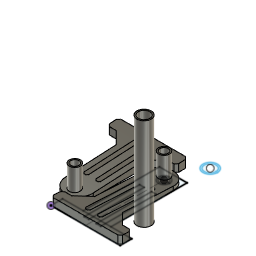
10lbs spool holder v3 (Autodesk Fusion 360 design; units mm, degrees)
Autodesk Fusion 360 part; units mm, degrees
sketch "Sketch1" plane through (0, 0, 0) normal (0, 0, 1) x (1, 0, 0) in component "Side"
  line L0 (0, 0) -> (150, 0)
  line L1 (75, 0) -> (75, 170) construction
  circle A0 centre (75, 170) radius 12
  circle A1 centre (75, 170) radius 9
  line L2 (150, 0) -> (150, 25)
  line L3 (0, 0) -> (0, 25)
  line L4 (0, 25) -> (150, 25)
  line L5 (45, 190) -> (105, 190)
  circle A2 centre (102.7681, 242.3233) radius 12.5
  circle A3 centre (102.7681, 242.3233) radius 15.5
  line L6 (45, 190) -> (45, 25)
  line L7 (105, 190) -> (105, 25)
  line L8 (57, 135) -> (67, 135)
  line L9 (67, 135) -> (67, 15)
  line L10 (67, 15) -> (57, 15)
  line L11 (57, 15) -> (57, 135)
  line L12 (93, 15) -> (93, 135)
  line L13 (93, 135) -> (83, 135)
  line L14 (83, 135) -> (83, 15)
  line L15 (83, 15) -> (93, 15)
  dimension "d1" = 150
  dimension "d2" = 170
  dimension "d3" = 24
  dimension "d4" = 18
  dimension "d5" = 25
  dimension "d6" = 25
  dimension "d9" = 60
  dimension "d10" = 190
  dimension "d11" = 25
  dimension "d16" = 25
  dimension "d17" = 31
  dimension "d20" = 45
  dimension "d28" = 10
  dimension "d29" = 120
  dimension "d30" = 15
  dimension "d31" = 8
  constraint coincident L0.start L3.start
  constraint horizontal L0
  constraint midpoint L0 L1.start
  constraint perpendicular L0 L1
  constraint coincident L1.end A0.centre
  constraint perpendicular L0 L2
  constraint perpendicular L0 L3
  constraint horizontal L4
  constraint perpendicular L1 L5
  constraint concentric A2 A3
  constraint coincident L4 L6.end
  constraint perpendicular L4 L6
  constraint coincident L4 L7.end
  constraint perpendicular L4 L7
  constraint horizontal L8
  constraint vertical L9
  constraint horizontal L10
  constraint vertical L11
  constraint symmetric L1 L8.start L12.end
  constraint symmetric L1 L8.end L13.end
  constraint symmetric L1 L9.end L14.end
  constraint symmetric L1 L10.end L12.start
  measures "d1" distance of L0.start L0.end
  measures "d2" distance of L1.start L1.end
  measures "d3" diameter of A0
  measures "d4" diameter of A1
  measures "d5" distance of L0.end L2.end
  measures "d6" distance of L0.start L3.end
  measures "d9" distance of L5.start L5.end
  measures "d10" distance of L0 L5
  measures "d11" distance of L0 L4
  measures "d16" diameter of A2
  measures "d17" diameter of A3
  measures "d20" distance of L3 L6
  measures "d28" distance of L8.start L8.end
  measures "d29" distance of L8.start L10.end
  measures "d30" distance of L0 L10
  measures "d31" distance of L1 L9
extrude "Extrude4" add sketch "Sketch1" along normal blind 10 contours L0 L2 L3 L4 L9 L10 L11 L12 L14 L15 | L4 L5 L6 L7 L8 L9 L11 L12 L13 L14 makes body 1 in component "Side"
draft "Draft1" angle -3 neutral plane through (93, 135, 0) pull (0, -1, 0) 1 faces at (15, 16.6667, 10) on bodies 1 in component "Side"
extrude "Extrude5" add sketch "Sketch1" along normal blind 55 contours A0 bodies 1 in component "Side"
chamfer "Chamfer1" distance 5 angle 45 4 edges at (0, 25, 7.8824) (0, 0, 8.5375) (150, 0, 8.5375) (150, 25, 7.8824) on bodies 1 in component "Side"
chamfer "Chamfer2" distance 25 angle 45 2 edges at (45, 25, 7.8824) (105, 25, 7.8824) on bodies 1 in component "Side"
fillet "Fillet1" radius 30 2 edges at (45, 190, 3.5588) (105, 190, 3.5588) on bodies 1 in component "Side"
chamfer "Chamfer3" distance 3 angle 45 8 edges at (93, 135, 5) (93, 15, 8.1445) (67, 15, 8.1445) (67, 135, 5) (83, 135, 5) (83, 15, 8.1445) (57, 15, 8.1445) (57, 135, 5) on bodies 1 in component "Side"
copy_body "CopyPasteBodies2" bodies 1 makes body 2 in component "Side"
move_body "Move2" bodies 2 to x (-1, 0, 0) y (0, -1, 0) z (0, 0, 1) at (76.008, 220.5643, 0) in component "Side"
extrude "Extrude6" add sketch "Sketch1" along normal blind 200 separate body contours A3 makes body 3 in component "Side"
move_body "Move3" bodies 3 to x (1, 0, 0) y (0, 1, 0) z (0, 0, 1) at (28.2686, -171.6106, 0) in component "Side"
extrude "Extrude1" [suppressed] in component "Side"
extrude "Extrude2" [suppressed] in component "Side"
copy_body "CopyPasteBodies1" [suppressed] in component "Side"
move_body "Move1" [suppressed] in component "Side"
extrude "Extrude3" [suppressed] in component "Side"
component "Side" placed x (1, 0, 0) y (0, 1, 0) z (0, 0, 1) at (0, 0, 0)
